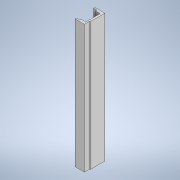
# Autodesk Inventor part: YaxisBalka
Saved by Autodesk Inventor 2020.1 (Build 241239000, 239)
## iProperties
Created: 2023-01-07
Part Number: YaxisBalka
Material: Типовые
Document SubType Name: Modeling
Designer: KirikDK
Density: 1 g/cm^3
Appearance: По умолчанию
Author: KirikDK
Autodesk Inventor part; units mm, degrees
ref_plane "YZ Plane" through (0, 0, 0) normal (1, 0, 0) x (0, 1, 0)
ref_plane "XZ Plane" through (0, 0, 0) normal (0, 1, 0) x (-1, 0, 0)
ref_plane "XY Plane" through (0, 0, 0) normal (0, 0, 1) x (1, 0, 0)
sketch "Эскиз1" plane through (0, 0, 0) normal (0, 1, 0) x (-1, 0, 0)
  line L0 (21.8182, 60) -> (-38.1818, 60)
  line L1 (-38.1818, 60) -> (-38.1818, -60)
  line L2 (-38.1818, -60) -> (21.8182, -60)
  line L3 (21.8182, -60) -> (21.8182, 60)
  line L4 (28, 44) -> (-26.1818, 44)
  line L5 (-26.1818, 44) -> (-26.1818, -44)
  line L6 (-26.1818, -44) -> (28, -44)
  line L7 (28, -44) -> (28, 44)
  line L8 (-38.1818, 60) -> (-34.1818, 60)
  line L9 (-34.1818, 60) -> (-34.1818, 28)
  line L10 (-34.1818, 28) -> (-38.1818, 28)
  line L11 (-38.1818, 28) -> (-38.1818, 60)
  line L12 (21.8182, -44) -> (1.8182, -44)
  line L13 (1.8182, -44) -> (1.8182, -52)
  line L14 (1.8182, -52) -> (21.8182, -52)
  line L15 (21.8182, -52) -> (21.8182, -44)
  line L16 (21.8182, 44) -> (1.8182, 44)
  line L17 (1.8182, 44) -> (1.8182, 52)
  line L18 (1.8182, 52) -> (21.8182, 52)
  line L19 (21.8182, 52) -> (21.8182, 44)
  point P0 (0, 0)
  point P1 (21.8182, -52)
  point P2 (1.8182, -44)
  dimension "d0" = 120
  dimension "d1" = 60
  dimension "d2" = 16
  dimension "d3" = 16
  dimension "d4" = 12
  dimension "d5" = 4
  dimension "d6" = 32
  dimension "d7" = 20
  dimension "d8" = 8
  dimension "d9" = 8
  dimension "d10" = 20
  constraints: 40 end point, 10 parallel, 5 horizontal, 5 perpendicular, 4 point on line
  measures "d0" distance of L0.end L1.end
  measures "d1" distance of L0.start L0.end
  measures "d2" distance between parallel lines of L0 L4
  measures "d3" distance between parallel lines of L2 L6
  measures "d4" distance between parallel lines of L1 L5
  measures "d5" distance of L9.end L10.end
  measures "d6" distance of L8.end L9.end
  measures "d7" distance between parallel lines of L19 L17
  measures "d8" distance between parallel lines of L0 L18
  measures "d9" distance between parallel lines of L2 L14
  measures "d10" distance between parallel lines of L3 L13
extrude "Выдавливание1" add sketch "Эскиз1" along normal blind 777 contours L3 L18 L17 L4 L5 L6 L13 L14 L2 L1 L10 L9 L0
